LED Light Battery Pack (Autodesk Fusion 360 design; units mm, degrees)
Autodesk Fusion 360 part; units mm, degrees
box "BoxPrimitive1" add length 103 width 64 height 22 placed x (0, 0, -1) y (-1, 0, 0) z (0, 1, 0) at (64, 0, 78) in component "Component"
sketch "Sketch2" plane through (0, 0, 0) normal (0, -1, 0) x (1, 0, 0) in component "Component"
  line L0 (0, -25) -> (64, -25)
  line L1 (64, -25) -> (64, 78)
  line L2 (64, 78) -> (0, 78)
  line L3 (0, 78) -> (0, -25)
  line L4 (39, -25) -> (24, -25)
  line L5 (24, -25) -> (24, -30)
  line L6 (24, -30) -> (39, -30)
  line L7 (39, -30) -> (39, -25)
  arc A0 (24, -30) -> (39, -30) centre (31.5, -26.9473) ccw
  constraint horizontal L4
  constraint vertical L5
  constraint horizontal L6
  constraint vertical L7
  constraint coincident L0 L4.start
extrude "Extrude1" add sketch "Sketch2" against normal blind 3 contours L0 L4 L5 L6 L7 | L6 A0 in component "Component"
sketch "Sketch3" plane through (0, 3, 0) normal (0, 1, 0) x (-1, 0, 0) in component "Component"
  arc A0 (-39, -30) -> (-24, -30) centre (-31.5, -26.9473) ccw
  line L0 (-24, -30) -> (-24, -25)
  line L1 (-24, -25) -> (-39, -25)
  line L2 (-39, -25) -> (-39, -30)
  line L3 (-27.5, -25) -> (-35.5, -25)
  line L4 (-35.5, -25) -> (-35.5, -29)
  line L5 (-35.5, -29) -> (-27.5, -29)
  line L6 (-27.5, -29) -> (-27.5, -25)
  arc A1 (-35.5, -29) -> (-27.5, -29) centre (-31.5, -26.0876) ccw
  constraint horizontal L3
  constraint vertical L4
  constraint horizontal L5
  constraint vertical L6
  constraint coincident L1 L3.start
extrude "Extrude2" cut sketch "Sketch3" against normal blind 5 contours L1 L3 L4 L5 L6 | L5 A1 in component "Component"
fillet "Fillet1" radius 2 1 edges at (0, 11, -25) in component "Component"
fillet "Fillet2" radius 2 1 edges at (0, 11, 78) in component "Component"
fillet "Fillet3" radius 2 1 edges at (64, 11, -25) in component "Component"
fillet "Fillet4" radius 2 1 edges at (64, 11, 78) in component "Component"
fillet "Fillet5" radius 2 8 edges at (0.5858, 22, 77.4142) (32, 22, 78) (63.4142, 22, 77.4142) (64, 22, 26.5) (63.4142, 22, -24.4142) (32, 22, -25) (0.5858, 22, -24.4142) (0, 22, 26.5) in component "Component"
sketch "Sketch1" plane through (0, 0, -25) normal (0, 0, -1) x (-1, 0, 0)
  line L0 (-2, 20) -> (-62, 20)
  line L1 (-62, 20) -> (-62, 0)
  line L2 (-62, 0) -> (-39, 0)
  line L3 (-39, 0) -> (-39, 3)
  line L4 (-39, 3) -> (-35.5, 3)
  line L5 (-35.5, 3) -> (-35.5, 0)
  line L6 (-35.5, 0) -> (-27.5, 0)
  line L7 (-27.5, 0) -> (-27.5, 3)
  line L8 (-27.5, 3) -> (-24, 3)
  line L9 (-24, 3) -> (-24, 0)
  line L10 (-24, 0) -> (-2, 0)
  line L11 (-2, 0) -> (-2, 20)
  circle A0 centre (-31.5187, 20) radius 7.4813
  constraint coincident L0 A0.centre
extrude "Extrude3" cut sketch "Sketch1" against normal blind 7 contours L0 A0 picked at (-33.0457, 17.6786) in component "Component"
pipe "Pipe1" cut diameter 6 along 1 edges at (31.5187, 20, -25) in component "Component"
sketch "Sketch2 (2)" plane through (0, 22, 0) normal (0, 1, 0) x (-1, 0, 0)
  line L0 (-2, 76) -> (-62, 76)
  line L1 (-62, 76) -> (-62, -23)
  line L2 (-24.0374, -23) -> (-2, -23)
  line L3 (-2, -23) -> (-2, 76)
  circle A0 centre (-31.0491, -11.1284) radius 11
  line L4 (-24.0374, -22.7639) -> (-24.0374, -23)
  line L5 (-62, -23) -> (-39, -23)
  line L6 (-39, -23) -> (-39, -22.7639)
  line L7 (-39, -22.7639) -> (-24.0374, -22.7639)
  dimension "d26" = 22
  measures "d26" diameter of A0
extrude "Extrude4" cut sketch "Sketch2 (2)" against normal blind 1 contours A0 in component "Component"
sketch "Sketch3 (2)" plane through (0, 21, 0) normal (0, 1, 0) x (-1, 0, 0)
  line L0 (-31.0491, -7.1059) -> (-31.0491, -15.1509) construction
  arc A0 (-30.1997, -15.9733) -> (-31.8985, -15.9733) centre (-31.0491, -11.1284) ccw
  arc A1 (-30.1997, -15.6907) -> (-31.8985, -15.6907) centre (-31.0491, -11.1284) ccw
  line L1 (-30.6514, -16.8752) -> (-30.6514, -13.4267)
  arc A2 (-30.6514, -13.4267) -> (-31.4468, -13.4267) centre (-31.0491, -13.4267) ccw
  line L2 (-31.4468, -13.4267) -> (-31.4468, -16.8752)
  arc A3 (-31.4468, -16.8752) -> (-30.6514, -16.8752) centre (-31.0491, -16.8752) ccw
  line L3 (-31.0491, -16.8752) -> (-31.0491, -13.4267) construction
  line L4 (-31.8985, -15.6907) -> (-31.8985, -15.9733)
  line L5 (-30.1997, -15.6907) -> (-30.1997, -15.9733)
  circle A4 centre (-31.0491, -11.1284) radius 11
  point P0 (-31.0491, -11.1284)
  point P1 (-31.0491, -15.1509)
  constraint concentric A0 A4
  constraint vertical L0
  constraint coincident P0 A0.centre
  constraint midpoint L0 P0
  constraint concentric A0 A1
  constraint tangent L1 A2
  constraint tangent A2 L2
  constraint parallel L1 L2
  constraint tangent L2 A3
  constraint tangent L1 A3
  constraint coincident L0 A2.centre
  constraint parallel L0 L3
  constraint coincident P1 L0.end
  constraint midpoint L3 P1
  constraint vertical L4
  constraint parallel L1 L5
extrude "Extrude5" cut sketch "Sketch3 (2)" against normal blind 0.5 contours A0 A1 L4 L5 | L1 A2 L2 A3 in component "Component"
component "Component" placed x (1, 0, 0) y (0, 1, 0) z (0, 0, 1) at (0, 0, 0)
